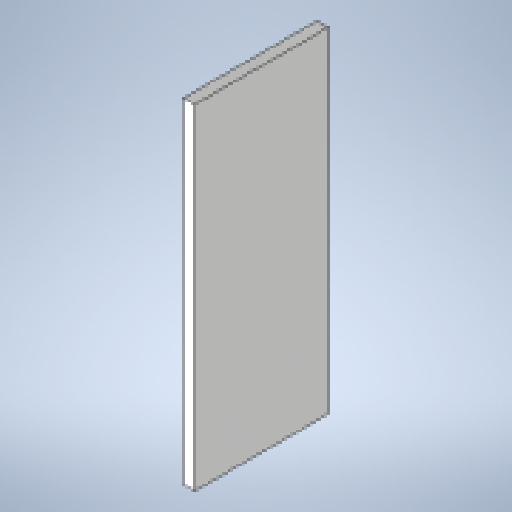
# Autodesk Inventor part: Top Plate
Saved by Autodesk Inventor 2023.4 (Build 274418000, 418)
## iProperties
Created: 2024-05-08
Part Number: Top Plate
Material: UHMW, White
Document SubType Name: Modeling
Designer: Nathan Cai
Mass: 10.8308 g
Surface Area: 81.0482 cm^2
Volume: 11.5222 cm^3
Density: 0.94 g/cm^3
Appearance: Smooth - White
Author: Nathan Cai
Autodesk Inventor part; units mm, degrees
ref_plane "YZ Plane" through (0, 0, 0) normal (1, 0, 0) x (0, 1, 0)
ref_plane "XZ Plane" through (0, 0, 0) normal (0, 1, 0) x (-1, 0, 0)
ref_plane "XY Plane" through (0, 0, 0) normal (0, 0, 1) x (1, 0, 0)
sketch "Sketch1" plane through (0, 0, 0) normal (1, 0, 0) x (0, 1, 0)
  line L0 (47.625, 19.05) -> (-47.625, 19.05)
  line L1 (-47.625, 19.05) -> (-47.625, -19.05)
  line L2 (-47.625, -19.05) -> (47.625, -19.05)
  line L3 (47.625, -19.05) -> (47.625, 19.05)
  line L4 (47.625, 19.05) -> (-47.625, -19.05) construction
  line L5 (-47.625, 19.05) -> (47.625, -19.05) construction
  point P0 (0, 0)
  dimension "d0" = 95.25
  dimension "d1" = 38.1
  constraints: 12 end point, 2 midpoint, 2 parallel, 1 horizontal, 1 perpendicular
  measures "d0" distance of L2.end L1.end
  measures "d1" distance of L1.end L0.end
extrude "Extrusion1" add sketch "Sketch1" along normal blind 3.175
body "Solid1"
